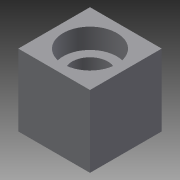
# Autodesk Inventor part: acmeBearingBlock
Saved by Autodesk Inventor 2013 (Build 170138000, 138)
## iProperties
Created: 2012-12-06
Part Number: acmeBearingBlock
Material: Generic
Document SubType Name: Modeling
Designer: Istvan
Density: 1 g/cm^3
Author: Istvan
Autodesk Inventor part; units mm, degrees
ref_plane "YZ Plane" through (0, 0, 0) normal (1, 0, 0) x (0, 1, 0)
ref_plane "XZ Plane" through (0, 0, 0) normal (0, 1, 0) x (-1, 0, 0)
ref_plane "XY Plane" through (0, 0, 0) normal (0, 0, 1) x (1, 0, 0)
sketch "Sketch1" plane through (0, 0, 0) normal (0, 1, 0) x (-1, 0, 0)
  line L0 (0, 0) -> (25.4, 0)
  line L1 (25.4, 0) -> (25.4, 25.4)
  line L2 (25.4, 25.4) -> (0, 25.4)
  line L3 (0, 25.4) -> (0, 0)
  dimension "d0" = 25.4
  dimension "d1" = 25.4
  constraints: 8 end point, 2 parallel, 1 horizontal, 1 perpendicular
  measures "d0" distance of L2.end L1.end
  measures "d1" distance of L1.end L0.end
extrude "Extrusion1" add sketch "Sketch1" along normal blind 12.7
sketch "Sketch2" plane through (0, 12.7, 0) normal (0, 1, 0) x (1, 0, 0)
  circle A0 centre (-12.7, -12.7) radius 9.525
  point P0 (-25.4, 0)
  dimension "d4" = 19.05
  dimension "d5" = 12.7
  dimension "d6" = 12.7
  constraints: 1 centre point
  measures "d4" diameter of A0
  measures "d5" horizontal distance of point (-25.4, 0) A0.centre
  measures "d6" horizontal distance of point (-25.4, 0) A0.centre
extrude "Extrusion2" cut sketch "Sketch2" against normal blind 7.1437
sketch "Sketch3" plane through (-12.7, 5.5563, 12.7) normal (0, 1, 0) x (1, 0, 0)
  circle A0 centre (0, 0) radius 9.525 projected
  circle A1 centre (0, 0) radius 3.175
  circle A2 centre (0, 0) radius 6.35
  point P0 (12.7, 12.7)
  dimension "d9" = 6.35
  dimension "d12" = 3.175
  dimension "d13" = 3.175
  constraints: 2 centre point, 2 coincident
  measures "d9" diameter of A1
  measures "d12" radial gap between concentric circles of A2 A1
  measures "d13" radial gap between concentric circles of A0 A2
extrude "Extrusion3" cut sketch "Sketch3" against normal through all contours A1 | A2
mirror "Mirror1" about plane through (-12.7, 0, 12.7) normal (0, -1, 0)
equation "\"d12\" = d13"
body "Solid1"
